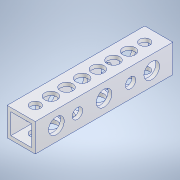
# Autodesk Inventor part: ハンド9x9_2
Saved by Autodesk Inventor 2020.3 (Build 243373000, 373)
## iProperties
Created: 2020-05-31
Part Number: ハンド9x9_2
Material: アルミニウム 6061
Document SubType Name: Modeling
Designer: totot
Mass: 3.35589 g
Surface Area: 25.4 cm^2
Volume: 1.24292 cm^3
Density: 2.7 g/cm^3
Appearance: アルミニウム - フラット
Author: totot
Autodesk Inventor part; units mm, degrees
ref_plane "YZ Plane" through (0, 0, 0) normal (1, 0, 0) x (0, 1, 0)
ref_plane "XZ Plane" through (0, 0, 0) normal (0, 1, 0) x (-1, 0, 0)
ref_plane "XY Plane" through (0, 0, 0) normal (0, 0, 1) x (1, 0, 0)
sketch "スケッチ1" plane through (0, 0, 0) normal (0, 0, 1) x (1, 0, 0)
  line L0 (0, 0) -> (9, 0)
  line L1 (9, 0) -> (9, -9)
  line L2 (9, -9) -> (0, -9)
  line L3 (0, -9) -> (0, 0)
  line L4 (1.2, -1.2) -> (7.8, -1.2)
  line L5 (7.8, -1.2) -> (7.8, -7.8)
  line L6 (7.8, -7.8) -> (1.2, -7.8)
  line L7 (1.2, -7.8) -> (1.2, -1.2)
  dimension "d0" = 9
  dimension "d1" = 9
  dimension "d2" = 1.2
  dimension "d3" = 1.2
  dimension "d4" = 1.2
  dimension "d5" = 1.2
  constraints: 16 end point, 4 parallel, 2 horizontal, 2 perpendicular
  measures "d0" distance of L1.end L2.end
  measures "d1" distance of L0.end L1.end
  measures "d2" distance between parallel lines of L0 L4
  measures "d3" distance between parallel lines of L3 L7
  measures "d4" distance between parallel lines of L2 L6
  measures "d5" distance between parallel lines of L1 L5
extrude "押し出し1" add sketch "スケッチ1" along normal blind 44
sketch "スケッチ2" plane through (0, 0, 0) normal (0, 1, 0) x (1, 0, 0)
  line L0 (0, 0) -> (0, -44) projected
  line L1 (9, 0) -> (0, 0) projected
  line L2 (0, -44) -> (9, -44) projected
  point P0 (4.5, -39.5)
  point P1 (4.5, -4.5)
  dimension "d8" = 4.5
  dimension "d26" = 4.5
  dimension "d27" = 4.5
  dimension "d28" = 4.5
  measures "d8" distance from line of L0 point (4.5, -39.5)
  measures "d26" distance from line of point (4.5, -39.5) L2
  measures "d27" distance from line of point (4.5, -4.5) L1
  measures "d28" distance from line of L0 point (4.5, -4.5)
hole "穴1" at (4.5, 0, 39.5) at (4.5, 0, 4.5) direction (0, -1, 0) diameter 3.3 end through all
sketch "スケッチ3" plane through (9, -9, 0) normal (1, 0, 0) x (0, 0, -1)
  line L0 (-44, 0) -> (-44, 9) projected
  line L1 (0, 9) -> (-44, 9) projected
  line L2 (0, 0) -> (0, 9) projected
  point P0 (-30.5, 4.5)
  point P1 (-13.5, 4.5)
  dimension "d17" = 13.5
  dimension "d18" = 4.5
  dimension "d29" = 13.5
  dimension "d30" = 4.5
  measures "d17" distance from line of L0 point (-30.5, 4.5)
  measures "d18" distance from line of point (-30.5, 4.5) L1
  measures "d29" distance from line of point (-13.5, 4.5) L2
  measures "d30" distance from line of L1 point (-13.5, 4.5)
hole "穴2" at (9, -4.5, 30.5) at (9, -4.5, 13.5) direction (-1, 0, 0) diameter 3.3 end through all
sketch "スケッチ4" plane through (0, -9, 0) normal (0, -1, 0) x (1, 0, 0)
  line L0 (9, 0) -> (9, 44) projected
  circle A0 centre (4.5, 39.5) radius 1.65 projected
  point P0 (0, 0)
  point P1 (4.5, 34.5)
  point P2 (4.5, 29.5)
  point P3 (4.5, 24.5)
  point P4 (4.5, 19.5)
  point P5 (4.5, 14.5)
  point P6 (4.5, 9.5)
  dimension "d31" = 4.5
  dimension "d32" = 5
  dimension "d35" = 5
  constraints: 1 vertical, 5 other
  measures "d31" distance from line of point (4.5, 34.5) L0
  measures "d32" distance of point (4.5, 34.5) A0.centre
  measures "d35" distance of point (4.5, 34.5) point (4.5, 29.5)
hole "穴3" at (4.5, -9, 34.5) at (4.5, -9, 29.5) at (4.5, -9, 24.5) at (4.5, -9, 19.5) at (4.5, -9, 14.5) at (4.5, -9, 9.5) direction (0, 1, 0) diameter 4 end through all
sketch "スケッチ5" plane through (0, -9, 0) normal (-1, 0, 0) x (0, 0, 1)
  circle A0 centre (13.5, 4.5) radius 1.65 projected
  line L0 (0, 9) -> (0, 0) projected
  line L1 (44, 9) -> (44, 0) projected
  line L2 (0, 9) -> (44, 9) projected
  circle A1 centre (30.5, 4.5) radius 1.65 projected
  point P0 (6.75, 4.5)
  point P1 (37.25, 4.5)
  point P2 (22, 4.5)
  dimension "d47" = 13.5
  dimension "d48" = 6.75
  dimension "d49" = 6.75
  dimension "d50" = 4.5
  dimension "d51" = 4.5
  dimension "d52" = 4.5
  dimension "d53" = 17
  dimension "d54" = 8.5
  measures "d47" distance from line of A0.centre L0
  measures "d48" distance from line of point (6.75, 4.5) L0
  measures "d49" distance from line of point (37.25, 4.5) L1
  measures "d50" distance from line of L2 point (37.25, 4.5)
  measures "d51" distance from line of L2 point (6.75, 4.5)
  measures "d52" distance from line of L2 point (22, 4.5)
  measures "d53" distance of A1.centre A0.centre
  measures "d54" distance of point (22, 4.5) A0.centre
hole "穴4" at (0, -4.5, 6.75) at (0, -4.5, 37.25) at (0, -4.5, 22) direction (1, 0, 0) diameter 5 end through all
equation "\"d3\" = d2"
equation "\"d4\" = d3"
equation "\"d5\" = d2"
equation "\"d26\" = d27"
equation "\"d28\" = d8"
equation "\"d29\" = d17"
equation "\"d30\" = d18"
equation "\"d48\" = 0.5 * d47"
equation "\"d49\" = d48"
equation "\"d51\" = d50"
equation "\"d52\" = d50"
equation "\"d54\" = 0.5 * d53"
